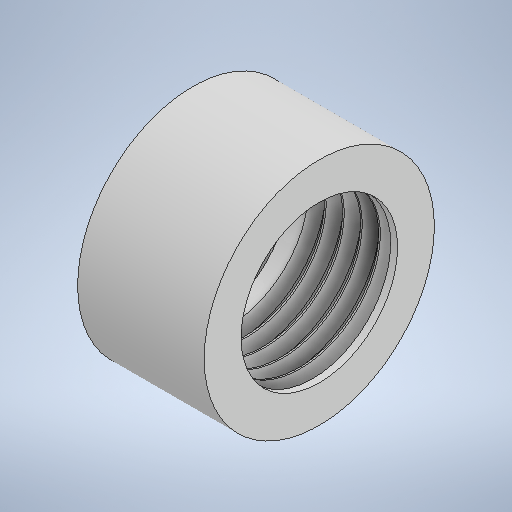
# Autodesk Inventor part: Innerer Differential Wurm Getriebe
Saved by Autodesk Inventor 2025.2 (Build 292293000, 293)
## iProperties
Created: 2024-11-22
Part Number: Innerer Differential Wurm Getriebe
Material: Generisch
Document SubType Name: Modeling
Designer: jensb
Density: 1 g/cm^3
Appearance: Vorgabe
Author: jensb
Autodesk Inventor part; units mm, degrees
ref_plane "YZ Plane" through (0, 0, 0) normal (1, 0, 0) x (0, 1, 0)
ref_plane "XZ Plane" through (0, 0, 0) normal (0, 1, 0) x (-1, 0, 0)
ref_plane "XY Plane" through (0, 0, 0) normal (0, 0, 1) x (1, 0, 0)
sketch "Skizze1" plane through (0, 0, 0) normal (0, 0, 1) x (1, 0, 0)
  line L0 (-27.5, 0) -> (27.5, 0)
  line L1 (-27.5, 34) -> (27.5, 34)
  line L2 (-27.5, 34) -> (-27.5, 50)
  line L3 (-27.5, 50) -> (27.5, 50)
  line L4 (27.5, 50) -> (27.5, 34)
  point P0 (0, 0)
  point P1 (0, 0)
  dimension "d0" = 68
  dimension "d1" = 100
  dimension "d2" = 55
  constraints: 10 end point, 2 horizontal, 2 perpendicular, 2 vertical alignment, 1 coincident, 1 midpoint, 1 vertical
  measures "d0" diameter of L1 L0
  measures "d1" diameter of L3 L0
  measures "d2" distance between parallel lines of L4 L2
revolve "Umdrehung1" add sketch "Skizze1" angle 360 about axis through (-27.5, 0, 0) along (1, 0, 0)
sketch "Skizze2" plane through (0, 0, 0) normal (0, 0, 1) x (1, 0, 0)
  arc A0 (26.4, -39.278) -> (28.6, -39.278) centre (27.5, -11.75) ccw
  line L0 (27.5, -23.5023) -> (27.5, -32.75) construction
  line L1 (27.5, -34) -> (27.5, 34) projected
  line L2 (30.15, -32.75) -> (24.85, -32.75) construction
  line L3 (27.5, -34) -> (-27.5, -34) projected
  line L4 (27.5, -34) -> (-27.5, -34) projected
  line L5 (26.4, -39.278) -> (23.9388, -34)
  line L6 (28.6, -39.278) -> (31.0612, -34)
  line L7 (31.0612, -34) -> (23.9388, -34)
  point P0 (0, 0)
  point P1 (27.5, 0)
  dimension "d4" = 27.55
  dimension "d5" = 2.2
  dimension "d9" = 11.75
  dimension "d10" = 21
  dimension "d11" = 5.3
  dimension "d21" = 25
  constraints: 10 end point, 3 vertical alignment, 2 point on circle, 1 centre point, 1 collinear, 1 horizontal, 1 horizontal alignment, 1 midpoint, 1 point on line, 1 vertical, 1 other
  measures "d4" radius of A0
  measures "d5" distance of L6.start L5.start
  measures "d9" vertical distance of point (0, 0) A0.centre
  measures "d10" distance from line of A0.centre L2
  measures "d11" distance of L2.start L2.end
  measures "d21" angle of L1 L5
coil "Spirale1" sketch "Skizze2" operation cut axis through (-10, 0, 0) along (-1, 0, 0) pitch 7.85 turns 5.095541 hand right
sketch "Skizze4" plane through (27.5, 0, 0) normal (1, 0, 0) x (0, 0, -1)
  circle A0 centre (0, 0) radius 50
  circle A1 centre (0, 0) radius 34
  point P0 (0, 0)
  constraints: 2 centre point, 2 coincident
extrude "Extrusion2" add sketch "Skizze4" against normal blind 3
sketch "Skizze5" plane through (-27.5, 0, 0) normal (-1, 0, 0) x (0, 0, 1)
  circle A0 centre (45, 0) radius 2.5
  circle A1 centre (0, 0) radius 45 construction
  circle A2 centre (22.5, 38.9711) radius 2.5
  circle A3 centre (-22.5, 38.9711) radius 2.5
  circle A4 centre (-45, 0) radius 2.5
  circle A5 centre (-22.5, -38.9711) radius 2.5
  circle A6 centre (22.5, -38.9711) radius 2.5
  point P0 (0, 0)
  dimension "d27" = 90
  dimension "d26" = 5
  dimension "d30" = 360
  constraints: 6 centre point, 2 horizontal alignment, 1 coincident, 15 other
  measures "d26" diameter of A0
extrude "Extrusion3" cut sketch "Skizze5" against normal blind 3
sketch "Skizze6" plane through (-27.5, 0, 0) normal (-1, 0, 0) x (0, 0, 1)
  circle A0 centre (0, 0) radius 41.5
  dimension "d35" = 83
  constraints: 1 centre point, 1 coincident
  measures "d35" diameter of A0
extrude "Extrusion4" cut sketch "Skizze6" against normal blind 8
